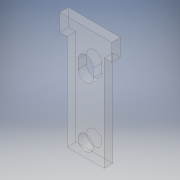
# Autodesk Inventor part: MotorMount
Saved by Autodesk Inventor 2018 (Build 220112000, 112)
## iProperties
Created: 2018-01-12
Part Number: MotorMount
Material: Polycarbonate, Clear
Document SubType Name: Modeling
Designer: Kyle
Density: 1.2 g/cm^3
Appearance: Polycarbonate - Clear
Author: Kyle
Autodesk Inventor part; units mm, degrees
ref_plane "YZ Plane" through (0, 0, 0) normal (1, 0, 0) x (0, 1, 0)
ref_plane "XZ Plane" through (0, 0, 0) normal (0, 1, 0) x (-1, 0, 0)
ref_plane "XY Plane" through (0, 0, 0) normal (0, 0, 1) x (1, 0, 0)
sketch "Sketch1" plane through (0, 0, 0) normal (0, 0, 1) x (1, 0, 0)
  line L0 (0, 0) -> (15.24, 0)
  line L1 (15.24, 0) -> (15.24, -5.08)
  line L2 (15.24, -5.08) -> (13.0175, -5.08)
  line L3 (13.0175, -5.08) -> (13.0175, -33.02)
  line L4 (0, 0) -> (0, -5.08)
  line L5 (0, -5.08) -> (2.2225, -5.08)
  line L6 (2.2225, -5.08) -> (2.2225, -33.02)
  line L7 (2.2225, -33.02) -> (13.0175, -33.02)
  circle A0 centre (7.62, -29.21) radius 2.2225
  line L8 (7.62, -6.985) -> (7.62, -6.985)
  line L9 (9.8425, -9.2075) -> (9.8425, -11.7475)
  line L10 (7.62, -13.97) -> (7.62, -13.97)
  line L11 (5.3975, -11.7475) -> (5.3975, -9.2075)
  arc A1 (9.8425, -9.2075) -> (7.62, -6.985) centre (7.62, -9.2075) ccw
  arc A2 (7.62, -6.985) -> (5.3975, -9.2075) centre (7.62, -9.2075) ccw
  arc A3 (5.3975, -11.7475) -> (7.62, -13.97) centre (7.62, -11.7475) ccw
  arc A4 (7.62, -13.97) -> (9.8425, -11.7475) centre (7.62, -11.7475) ccw
  point P0 (9.8425, -13.97)
  point P1 (9.8425, -6.985)
  dimension "d0" = 15.24
  dimension "d1" = 5.08
  dimension "d2" = 2.2225
  dimension "d3" = 27.94
  dimension "d4" = 2.2225
  dimension "d5" = 4.445
  dimension "d6" = 3.81
  dimension "d7" = 6.985
  dimension "d8" = 6.985
  dimension "d9" = 2.2225
  constraints: 24 end point, 8 point on circle, 8 tangent, 5 centre point, 4 point on line, 4 vertical, 3 equal radius, 3 horizontal, 3 perpendicular, 2 parallel
  measures "d0" distance of L0.start L0.end
  measures "d1" distance of L0.end L1.end
  measures "d2" distance of L1.end L2.end
  measures "d3" distance of L2.end L3.end
  measures "d4" distance of L4.end L5.end
  measures "d5" diameter of A0
  measures "d6" distance from line of L7 A0.centre
  measures "d7" distance of point (9.843, -6.985) point (9.843, -13.97)
  measures "d8" distance between parallel lines of L0 L8
  measures "d9" radius of A1
extrude "Extrusion1" add sketch "Sketch1" along normal blind 2.54
body "Solid1"
